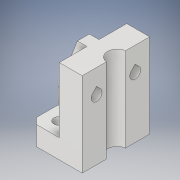
# Autodesk Inventor part: Piston Smooth rod holder
Saved by Autodesk Inventor 2018 (Build 220112000, 112)
## iProperties
Created: 2013-10-18
Part Number: Piston Smooth rod holder
Material: ASA Plastic
Document SubType Name: Modeling
Designer: Gabriel Smolnycki
Mass: 12.6588 g
Surface Area: 48.9866 cm^2
Volume: 11.8307 cm^3
Density: 1.07 g/cm^3
Appearance: Smooth - White ASA
Sending System: SolidWorks 2017
Last Author: Gabriel Smolnycki
Last Saved: 2017-09-14
Author: Gabriel Smolnycki
Autodesk Inventor part; units mm, degrees
ref_plane "YZ Plane" through (0, 0, 0) normal (1, 0, 0) x (0, 1, 0)
ref_plane "XZ Plane" through (0, 0, 0) normal (0, 1, 0) x (-1, 0, 0)
sketch "Sketch1" plane through (0, 0, 0) normal (0, 1, 0) x (-1, 0, 0)
  line L0 (22, -14) -> (0.5, -14)
  line L1 (0.5, -14) -> (0.5, 14)
  line L2 (22, 14) -> (0.5, 14)
  line L3 (22, 14) -> (22, -14)
  constraints: 8 end point, 2 horizontal, 2 vertical
extrude "Extrusion5" add sketch "Sketch1" along normal blind 35
sketch "Sketch2" plane through (-22, 0, -14) normal (-1, 0, 0) x (0, 0, 1)
  line L0 (28, 35) -> (16.5, 35)
  line L1 (16.5, 8) -> (16.5, 35)
  line L2 (28, 35) -> (28, 8)
  line L3 (28, 8) -> (16.5, 8)
  constraints: 8 end point, 2 horizontal, 2 vertical
extrude "Extrusion4" cut sketch "Sketch2" against normal blind 12 draft 0
sketch "Sketch3" plane through (-22, 0, -14) normal (-1, 0, 0) x (0, 0, 1)
  line L0 (11.5, 8) -> (11.5, 35)
  line L1 (0, 35) -> (0, 8)
  line L2 (11.5, 8) -> (0, 8)
  line L3 (11.5, 35) -> (0, 35)
  constraints: 8 end point, 2 horizontal, 2 vertical
extrude "Extrusion3" cut sketch "Sketch3" against normal blind 12 draft 0
chamfer "Chamfer3" distance 21 angle 20.854 1 edges at (-22, 35, 0) measured on face at (-22, 2.6667, -0.8333)
chamfer "Chamfer2" distance 2.5 angle 45 1 edges at (-22, 4, 14)
chamfer "Chamfer1" distance 2.5 angle 45 1 edges at (-22, 4, -14)
ref_plane "Work Plane1" through (0, 0, 0) normal (-0.9921567, 0, 0.125) x (0, 1, 0)
sketch "Sketch4" plane through (0, 0, 0) normal (-0.9921567, 0, 0.125) x (0, 1, 0)
  line L0 (0, 4) -> (35, 4)
  line L1 (0, 4) -> (0, 0)
  line L2 (35, 4) -> (35, 0)
  line L3 (0, 0) -> (35, 0)
  line L4 (0, 0) -> (10, 0)
  constraints: 10 end point, 3 horizontal, 2 vertical
revolve "Revolution1" cut sketch "Sketch4" angle 165.638 about axis through (0, 0, 0) along (0, 1, 0)
hole "Hole2" at (-16, 0, 8) direction (0, 1, 0) diameter 4.5 depth 8
sketch "Sketch5" plane through (0, 0, 0) normal (0, 1, 0) x (-1, 0, 0)
  point P0 (16, 8)
hole "Hole1" at (-16, 0, -8) direction (0, 1, 0) diameter 4.5 depth 8
sketch "Sketch7" plane through (-10, 0, -14) normal (-1, 0, 0) x (0, 0, 1)
  arc A0 (4.409, 26.591) -> (7.591, 26.591) centre (6, 25) ccw
  line L0 (6, 28.182) -> (4.409, 26.591)
  line L1 (7.591, 26.591) -> (6, 28.182)
  constraints: 4 end point, 2 perpendicular, 2 point on circle, 1 centre point
extrude "Extrusion2" cut sketch "Sketch7" against normal blind 9.5
sketch "Sketch8" plane through (-10, 0, -14) normal (-1, 0, 0) x (0, 0, 1)
  line L0 (22, 28.182) -> (20.409, 26.591)
  line L1 (23.591, 26.591) -> (22, 28.182)
  arc A0 (20.409, 26.591) -> (23.591, 26.591) centre (22, 25) ccw
  constraints: 4 end point, 2 perpendicular, 2 point on circle, 1 centre point
extrude "Extrusion1" cut sketch "Sketch8" against normal blind 9.5
sketch "Sketch6" plane through (0, 0, 0) normal (0, 1, 0) x (-1, 0, 0)
  point P0 (16, -8)
body "Solid3"
